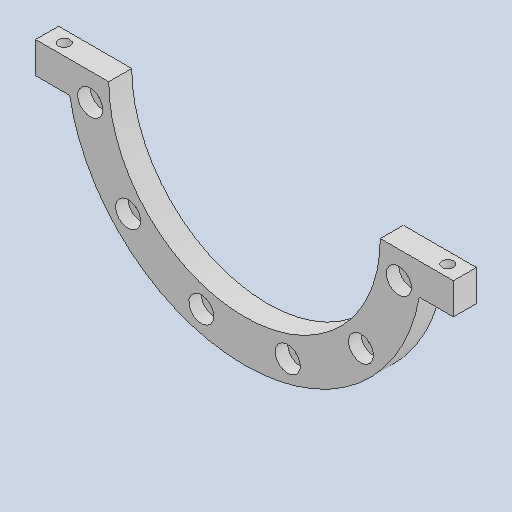
# Autodesk Inventor part: ДМФ 093 Постель КОРМА v2.0
Saved by Autodesk Inventor 2026.2 (Build 302298000, 298)
## iProperties
Created: 2024-04-28
Part Number: ДМФ 093 Постель КОРМА v2.0
Material: Nylon 6
Document SubType Name: Sheet Metal
Designer: admin
Density: 1.12 g/cm^3
Appearance: Default
Stock Number: Постель_Корма
Sheet Metal Rule: Default
Sheet Metal Width: 0,000 mm
Sheet Metal Length: 0,000 mm
Sheet Metal Area: 0,000 mm^2
Author: pokla
Autodesk Inventor part; units mm, degrees
ref_plane "YZ Plane" through (0, 0, 0) normal (1, 0, 0) x (0, 1, 0)
ref_plane "XZ Plane" through (0, 0, 0) normal (0, 1, 0) x (-1, 0, 0)
ref_plane "XY Plane" through (0, 0, 0) normal (0, 0, 1) x (1, 0, 0)
sketch "Sketch1" plane through (0, 0, 0) normal (0, 0, 1) x (1, 0, 0)
  circle A0 centre (0, 0) radius 150 construction
  line L0 (0, 150) -> (0, 170) construction
  line L1 (0, 150) -> (0, 130) construction
  circle A1 centre (0, 0) radius 130
  circle A2 centre (0, 0) radius 170
  line L2 (-130, 0) -> (-130, 80) construction
  line L3 (-130, 80) -> (-170, 80) construction
  line L4 (-170, 80) -> (-170, 0) construction
  line L5 (-130, 0) -> (-170, 0)
  line L6 (-170, 0) -> (-200, 0)
  line L7 (-200, 0) -> (-200, -30)
  line L8 (-200, -30) -> (-167.332, -30)
  line L9 (-1.5, -168) -> (1.5, -168)
  line L10 (1.5, -168) -> (1.5, -210)
  line L11 (1.5, -210) -> (-1.5, -210)
  line L12 (-1.5, -210) -> (-1.5, -168)
  line L13 (0, -168) -> (0, -130)
  line L14 (-1.5, -210) -> (-30, -210)
  line L15 (-30, -210) -> (-30, -167.332)
  line L16 (0, -168) -> (0, -170)
  point P0 (170, 0)
  point P1 (0, -210)
  point P2 (-1.5, -169.9934)
  point P3 (1.5, -169.9934)
  dimension "d26" = 80
  dimension "d36" = 40
  dimension "d40" = 30
  dimension "d41" = 30
  dimension "d74" = 260
  dimension "d75" = 3
  dimension "d76" = 42
  dimension "d77" = 30
  dimension "d78" = 2
  constraints: 34 end point, 9 point on circle, 6 perpendicular, 5 vertical, 3 coincident, 3 horizontal, 2 centre point, 2 midpoint, 2 parallel, 2 tangent, 2 vertical alignment, 1 collinear, 1 line through centre, 1 point on line, 2 other
  measures "d26" distance of L2.start L2.end
  measures "d36" distance of L1.end L0.end
  measures "d40" distance of L4.end L6.end
  measures "d41" distance of L6.end L7.end
  measures "d74" diameter of A1
  measures "d75" distance of L9.start L9.end
  measures "d76" distance of L11.end L9.start
  measures "d77" distance from line of point (0, -210) L15
  measures "d78" distance of L13.start L16.end
extrude "Extrusion1" add sketch "Sketch1" against normal blind 22 contours A1 L13 L9 L12 A2 L5 | A2 L8 L7 L6 | L16 A2 L12 L9
sketch "Sketch10" plane through (-200, -30, 0) normal (0, -1, 0) x (1, 0, 0)
  line L0 (0, 0) -> (32.668, 0) projected
  line L1 (0, 0) -> (0, -22) projected
  line L2 (32.668, -22) -> (0, -22) projected
  line L3 (32.668, 0) -> (32.668, -22) projected
  circle A0 centre (16.334, -11) radius 5.5
  line L4 (0, 0) -> (0, -22) projected
  line L5 (0, 0) -> (32.668, 0) projected
  point P0 (200, 0)
  point P1 (0, -11)
  point P2 (16.334, 0)
  dimension "d79" = 11
  constraints: 2 midpoint, 1 centre point, 1 horizontal alignment, 1 vertical alignment
  measures "d79" diameter of A0
extrude "Extrusion9" cut sketch "Sketch10" against normal through all contours A0
mirror "Mirror3" about plane through (0, 0, 0) normal (1, 0, 0) of "Extrusion1", "Extrusion9"
sketch "Sketch12" plane through (0, 0, 0) normal (0, 0, 1) x (1, 0, 0)
  line L0 (0, 0) -> (-150, 0) construction
  line L1 (0, 0) -> (-147.7212, -26.0472) construction
  circle A0 centre (0, 0) radius 150 construction
  dimension "d86" = 10
  dimension "d87" = 300
  constraints: 4 end point, 2 coincident, 2 point on circle, 1 centre point, 1 horizontal
  measures "d86" angle of L1 L0
  measures "d87" diameter of A0
hole "Hole4" at (-147.7212, -26.0472, 0) direction (0, 0, -1) diameter 11 end through all counterbore diameter 24 counterbore depth 12
pattern_circular "Circular Pattern5" count 6 over 160 about axis through (0, 0, -10) along (0, 0, 1) of "Hole4"
equation "\"d41\" = d40"
equation "\"d77\" = d41"
equation "\"d93\" = Thickness"
equation "\"BendReliefDepth\" = 0.5 * Thickness"
equation "\"Thickness\" = 30"
body "Solid1"
